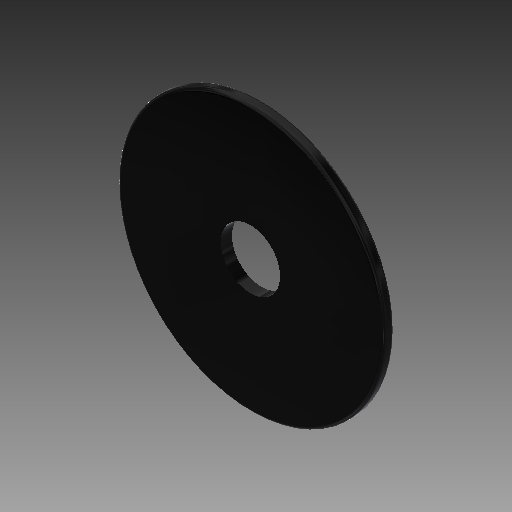
# Autodesk Inventor part: JLF-TP-8YT_ring
Saved by Autodesk Inventor 2019 (Build 230136000, 136)
## iProperties
Created: 2013-01-27
Part Number: JLF-TP-8YT_ring
Material: ABS Plastic
Document SubType Name: Modeling
Designer: xylzlyx
Density: 1 g/cm^3
Appearance: Smooth - White
Author: xylzlyx
Autodesk Inventor part; units mm, degrees
ref_plane "YZ Plane" through (0, 0, 0) normal (1, 0, 0) x (0, 1, 0)
ref_plane "XZ Plane" through (0, 0, 0) normal (0, 1, 0) x (-1, 0, 0)
ref_plane "XY Plane" through (0, 0, 0) normal (0, 0, 1) x (1, 0, 0)
sketch "Sketch" plane through (0, 0, 0) normal (0, 0, 1) x (1, 0, 0)
  circle A0 centre (0, 0) radius 4
  circle A1 centre (0, 0) radius 18
  dimension "d0" = 8
  dimension "d1" = 36
  constraints: 2 centre point, 2 coincident
  measures "d0" diameter of A0
  measures "d1" diameter of A1
extrude "Ring" add sketch "Sketch" along normal blind 1.5
fillet "Fillet1" radius 0.5 2 edges at (-18, 0, 1.5) (-18, 0, 0)
body "Solid1"
